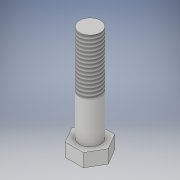
# Autodesk Inventor part: 3 8t 1 1 2 bolt
Saved by Autodesk Inventor 2018 (Build 220112000, 112)
## iProperties
Created: 2019-03-20
Part Number: 3 8t 1 1 2 bolt
Material: Generic
Document SubType Name: Modeling
Designer: S-4008082
Density: 1 g/cm^3
Appearance: Default
Author: S-4008082
Autodesk Inventor part; units mm, degrees
ref_plane "YZ Plane" through (0, 0, 0) normal (1, 0, 0) x (0, 1, 0)
ref_plane "XZ Plane" through (0, 0, 0) normal (0, 1, 0) x (-1, 0, 0)
ref_plane "XY Plane" through (0, 0, 0) normal (0, 0, 1) x (1, 0, 0)
sketch "Sketch1" plane through (0, 0, 0) normal (0, 1, 0) x (-1, 0, 0)
  circle A0 centre (0, 0) radius 4.7625
  dimension "d0" = 9.525
  constraints: 1 centre point, 1 coincident
  measures "d0" diameter of A0
extrude "Extrusion1" add sketch "Sketch1" along normal blind 27.1272
thread "Thread1" size "3/8-16 UNC" class "2A" standard "ANSI Unified Screw Threads" length 25.4
sketch "Sketch2" plane through (0, 0, 0) normal (0, -1, 0) x (1, 0, 0)
  circle A0 centre (0, 0) radius 4.7625
  constraints: 1 centre point, 1 coincident
extrude "Extrusion2" add sketch "Sketch2" along normal blind 16.5608
sketch "Sketch3" plane through (0, -16.5608, 0) normal (0, -1, 0) x (1, 0, 0)
  circle A0 centre (0, 0) radius 4.7625 projected
  line L0 (-4.0988, -7.0993) -> (-8.1976, 0)
  line L1 (-8.1976, 0) -> (-4.0988, 7.0993)
  line L2 (-4.0988, 7.0993) -> (4.0988, 7.0993)
  line L3 (4.0988, 7.0993) -> (8.1976, 0)
  line L4 (8.1976, 0) -> (4.0988, -7.0993)
  line L5 (4.0988, -7.0993) -> (-4.0988, -7.0993)
  dimension "d9" = 14.1986
  dimension "d10" = 14.1986
  constraints: 12 end point, 1 coincident, 13 other
  measures "d9" distance between parallel lines of L2 L5
  measures "d10" distance between parallel lines of L0 L3
extrude "Extrusion3" add sketch "Sketch3" along normal blind 5.969 contours A0 | L0 L1 L2 L3 L4 L5
body "Solid1"
